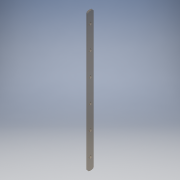
# Autodesk Inventor part: ArmSpacer6
Saved by Autodesk Inventor 2019 (Build 230136000, 136)
## iProperties
Created: 2019-01-14
Part Number: ArmSpacer6
Material: Polycarbonate, Smoke
Document SubType Name: Modeling
Designer: nxgam
Density: 1.2 g/cm^3
Appearance: Polycarbonate - Smoked
Author: nxgam
Autodesk Inventor part; units mm, degrees
ref_plane "YZ Plane" through (0, 0, 0) normal (1, 0, 0) x (0, 1, 0)
ref_plane "XZ Plane" through (0, 0, 0) normal (0, 1, 0) x (-1, 0, 0)
ref_plane "XY Plane" through (0, 0, 0) normal (0, 0, 1) x (1, 0, 0)
sketch "Sketch1" plane through (0, 0, 0) normal (1, 0, 0) x (0, 1, 0)
  line L0 (3.175, 0) -> (240.665, 0)
  line L1 (243.84, -3.175) -> (243.84, -6.985)
  line L2 (240.665, -10.16) -> (3.175, -10.16)
  line L3 (0, -6.985) -> (0, -3.175)
  arc A0 (243.84, -3.175) -> (240.665, 0) centre (240.665, -3.175) ccw
  arc A1 (240.665, -10.16) -> (243.84, -6.985) centre (240.665, -6.985) ccw
  arc A2 (3.175, 0) -> (0, -3.175) centre (3.175, -3.175) ccw
  arc A3 (0, -6.985) -> (3.175, -10.16) centre (3.175, -6.985) ccw
  line L4 (0, -5.08) -> (243.84, -5.08) construction
  point P0 (0, 0)
  point P1 (243.84, -10.16)
  point P2 (243.84, 0)
  point P3 (0, -10.16)
  point P4 (20.32, -5.08)
  point P5 (60.96, -5.08)
  point P6 (101.6, -5.08)
  point P7 (142.24, -5.08)
  point P8 (182.88, -5.08)
  point P9 (223.52, -5.08)
  dimension "d0" = 243.84
  dimension "d1" = 10.16
  dimension "d2" = 3.175
  dimension "d3" = 20.32
  dimension "d6" = 40.64
  dimension "d21" = 101.6
  constraints: 10 end point, 9 point on line, 8 point on circle, 8 tangent, 4 centre point, 3 equal radius, 2 horizontal, 2 midpoint, 2 parallel, 1 perpendicular, 5 other
  measures "d0" distance of point (243.84, -10.16) point (0, -10.16)
  measures "d1" distance of point (243.84, 0) point (243.84, -10.16)
  measures "d2" radius of A0
  measures "d3" distance of L4.start point (20.32, -5.08)
  measures "d6" distance of point (20.32, -5.08) point (60.96, -5.08)
  measures "d21" distance from line of L1 point (142.24, -5.08)
extrude "Extrusion1" add sketch "Sketch1" along normal blind 2.794
hole "Hole3" at (0, 20.32, -5.08) at (0, 60.96, -5.08) at (0, 101.6, -5.08) at (0, 142.24, -5.08) at (0, 182.88, -5.08) at (0, 223.52, -5.08) direction (1, 0, 0) diameter 4 end through all
body "Solid1"
